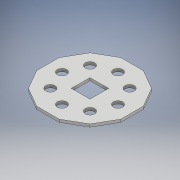
# Autodesk Inventor part: P2-11
Saved by Autodesk Inventor 2017 (Build 210142000, 142)
## iProperties
Created: 2017-02-09
Part Number: P2-11
Material: Generic
Document SubType Name: Modeling
Designer: Schaffel
Density: 1 g/cm^3
Appearance: Default
Author: Schaffel
Autodesk Inventor part; units mm, degrees
ref_plane "YZ Plane" through (0, 0, 0) normal (1, 0, 0) x (0, 1, 0)
ref_plane "XZ Plane" through (0, 0, 0) normal (0, 1, 0) x (-1, 0, 0)
ref_plane "XY Plane" through (0, 0, 0) normal (0, 0, 1) x (1, 0, 0)
sketch "Sketch1" plane through (0, 0, 0) normal (0, 0, 1) x (1, 0, 0)
  line L0 (65.8846, 0) -> (24.1154, 24.1154)
  line L1 (24.1154, 24.1154) -> (0, 65.8846)
  line L2 (0, 65.8846) -> (0, 114.1154)
  line L3 (0, 114.1154) -> (24.1154, 155.8846)
  line L4 (24.1154, 155.8846) -> (65.8846, 180)
  line L5 (65.8846, 180) -> (114.1154, 180)
  line L6 (114.1154, 180) -> (155.8846, 155.8846)
  line L7 (155.8846, 155.8846) -> (180, 114.1154)
  line L8 (180, 114.1154) -> (180, 65.8846)
  line L9 (180, 65.8846) -> (155.8846, 24.1154)
  line L10 (155.8846, 24.1154) -> (114.1154, 0)
  line L11 (114.1154, 0) -> (65.8846, 0)
  line L12 (70, 70) -> (110, 70)
  line L13 (110, 70) -> (110, 110)
  line L14 (110, 110) -> (70, 110)
  line L15 (70, 110) -> (70, 70)
  circle A0 centre (90, 150) radius 10
  circle A1 centre (47.5736, 132.4264) radius 10
  circle A2 centre (132.4264, 132.4264) radius 10
  circle A3 centre (150, 90) radius 10
  circle A4 centre (30, 90) radius 10
  circle A5 centre (47.5736, 47.5736) radius 10
  circle A6 centre (90, 30) radius 10
  circle A7 centre (132.4264, 47.5736) radius 10
  point P0 (0, 0)
  point P1 (90, 90)
  point P2 (90, 90)
  dimension "d1" = 20
  dimension "d2" = 20
  constraints: 32 end point, 8 centre point, 3 perpendicular, 1 horizontal, 25 other
  measures "d1" diameter of A1
  measures "d2" diameter of A2
extrude "Extrusion1" add sketch "Sketch1" along normal blind 6
body "Solid1"
